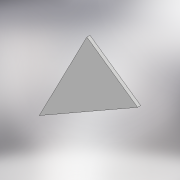
# Autodesk Inventor part: 1
Saved by Autodesk Inventor 2020 (Build 240168000, 168)
## iProperties
Created: 2019-05-26
Part Number: 1
Material: Generic
Document SubType Name: Modeling
Designer: chitl
Density: 1 g/cm^3
Appearance: Default
Author: chitl
Autodesk Inventor part; units mm, degrees
ref_plane "YZ Plane" through (0, 0, 0) normal (1, 0, 0) x (0, 1, 0)
ref_plane "XZ Plane" through (0, 0, 0) normal (0, 1, 0) x (-1, 0, 0)
ref_plane "XY Plane" through (0, 0, 0) normal (0, 0, 1) x (1, 0, 0)
sketch "Sketch1" plane through (0, 0, 0) normal (0, 0, 1) x (1, 0, 0)
  line L0 (124.8783, 71.1673) -> (166.7462, -5.9795)
  line L1 (166.7462, -5.9795) -> (-1.0811, -0.8611)
  line L2 (-1.0811, -0.8611) -> (124.8783, 71.1673)
  line L3 (59.8785, 116.6907) -> (124.8783, 71.1673)
  line L4 (59.8785, 116.6907) -> (-1.0811, -0.8611)
  point P0 (0, 0)
  constraints: 10 end point
extrude "Extrusion1" add sketch "Sketch1" along normal blind 4 contours L2 L4 L3
body "Solid1"
